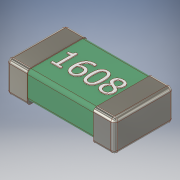
# Autodesk Inventor part: Resistor_1608-0.5mm
Saved by Autodesk Inventor 2018 (Build 220112000, 112)
## iProperties
Created: 2016-08-15
Part Number: Resistor_1608-0.5mm
Material: Copper
Document SubType Name: Modeling
Designer: Bradley
Density: 8.94 g/cm^3
Appearance: Copper - Satin
Author: Bradley
Autodesk Inventor part; units mm, degrees
ref_plane "YZ Plane" through (0, 0, 0) normal (1, 0, 0) x (0, 1, 0)
ref_plane "XZ Plane" through (0, 0, 0) normal (0, 1, 0) x (-1, 0, 0)
ref_plane "XY Plane" through (0, 0, 0) normal (0, 0, 1) x (1, 0, 0)
sketch "Sketch1" plane through (0, 0, 0) normal (0, 0, 1) x (1, 0, 0)
  line L0 (-0.775, 0.4) -> (-0.475, 0.4)
  line L1 (-0.475, 0.4) -> (-0.475, -0.05)
  line L2 (-0.475, -0.05) -> (-0.775, -0.05)
  line L3 (-0.775, -0.05) -> (-0.775, 0.4)
  line L4 (-0.475, 0.39) -> (0.475, 0.39)
  line L5 (0.475, 0.39) -> (0.475, 0)
  line L6 (0.475, 0) -> (-0.475, 0)
  line L7 (-0.475, 0) -> (-0.475, 0.39)
  line L8 (0.475, 0.4) -> (0.775, 0.4)
  line L9 (0.775, 0.4) -> (0.775, -0.05)
  line L10 (0.775, -0.05) -> (0.475, -0.05)
  line L11 (0.475, -0.05) -> (0.475, 0.4)
  point P0 (0, 0)
  point P1 (0, 0.39)
  point P2 (0, 0)
  dimension "d0" = 1.55
  dimension "d1" = 0.45
  dimension "d2" = 0.3
  dimension "d3" = 0.05
  dimension "d6" = 0.01
  constraints: 24 end point, 6 parallel, 3 horizontal, 3 perpendicular, 3 point on line, 2 collinear, 2 midpoint, 1 coincident, 1 vertical alignment
  measures "d0" distance between parallel lines of L9 L3
  measures "d1" distance of L2.end L0.start
  measures "d2" distance of L1.end L2.end
  measures "d3" distance between parallel lines of L2 L6
  measures "d6" distance between parallel lines of L4 L0
extrude "Extrusion1" add sketch "Sketch1" along normal mid plane 0.85 contours L0 L1 L2 L3 | L11 L8 L9 L10 L5
extrude "Extrusion2" add sketch "Sketch1" along normal mid plane 0.84 contours L4 L5 L6 L1
sketch "Sketch3" plane through (-0.475, 0.39, 0.42) normal (0, 1, 0) x (1, 0, 0)
  line L0 (0, 0) -> (0, 0.84) projected
  line L1 (0.95, 0) -> (0, 0) projected
  line L2 (0.95, 0.84) -> (0.95, 0) projected
  line L3 (0, 0.84) -> (0.95, 0.84) projected
  line L4 (0.95, 0.845) -> (0.95, -0.005) construction
  line L5 (0.95, 0.2582) -> (0, 0.2582) construction
  line L6 (0, 0.845) -> (0, -0.005) construction
  line L7 (0.2166, 0.2582) -> (0.0702, 0.2582)
  line L8 (0.0702, 0.2582) -> (0.0702, 0.2888)
  line L9 (0.0702, 0.2888) -> (0.1247, 0.2888)
  line L10 (0.1247, 0.2888) -> (0.1247, 0.4899)
  line L11 (0.1247, 0.4899) -> (0.0702, 0.4899)
  line L12 (0.0702, 0.4899) -> (0.0702, 0.5174)
  spline S0 degree 2 poles (0.0702, 0.5174) (0.1011, 0.5174) (0.1303, 0.5349) (0.1322, 0.5592) knots 0 0 0 1 2 2 2
  line L13 (0.1322, 0.5592) -> (0.1633, 0.5592)
  line L14 (0.1633, 0.5592) -> (0.1633, 0.2888)
  line L15 (0.1633, 0.2888) -> (0.2166, 0.2888)
  line L16 (0.2166, 0.2888) -> (0.2166, 0.2582)
  spline S1 degree 2 poles (0.4614, 0.3555) (0.4614, 0.3324) (0.4461, 0.2932) (0.4332, 0.2801) knots 0 0 0 1 2 2 2
  spline S2 degree 2 poles (0.4332, 0.2801) (0.4198, 0.2662) (0.3863, 0.2519) (0.3661, 0.2519) knots 0 0 0 1 2 2 2
  spline S3 degree 2 poles (0.3661, 0.2519) (0.3459, 0.2519) (0.3126, 0.2655) (0.3, 0.2791) knots 0 0 0 1 2 2 2
  spline S4 degree 2 poles (0.3, 0.2791) (0.2844, 0.2954) (0.2669, 0.3501) (0.2669, 0.39) knots 0 0 0 1 2 2 2
  spline S5 degree 2 poles (0.2669, 0.39) (0.2669, 0.4291) (0.2829, 0.4921) (0.2997, 0.5154) knots 0 0 0 1 2 2 2
  spline S6 degree 2 poles (0.2997, 0.5154) (0.316, 0.5383) (0.3675, 0.5638) (0.4013, 0.5638) knots 0 0 0 1 2 2 2
  spline S7 degree 2 poles (0.4013, 0.5638) (0.4113, 0.5638) (0.4288, 0.5619) (0.4354, 0.5597) knots 0 0 0 1 2 2 2
  line L17 (0.4354, 0.5597) -> (0.4354, 0.521)
  line L18 (0.4354, 0.521) -> (0.4337, 0.521)
  spline S8 degree 2 poles (0.4337, 0.521) (0.4281, 0.5239) (0.4077, 0.529) (0.396, 0.529) knots 0 0 0 1 2 2 2
  spline S9 degree 2 poles (0.396, 0.529) (0.3585, 0.529) (0.3126, 0.4785) (0.3082, 0.4289) knots 0 0 0 1 2 2 2
  spline S10 degree 2 poles (0.3082, 0.4289) (0.3226, 0.4388) (0.3527, 0.4498) (0.3707, 0.4498) knots 0 0 0 1 2 2 2
  spline S11 degree 2 poles (0.3707, 0.4498) (0.3882, 0.4498) (0.4145, 0.4427) (0.4288, 0.432) knots 0 0 0 1 2 2 2
  spline S12 degree 2 poles (0.4288, 0.432) (0.4453, 0.4196) (0.4614, 0.3812) (0.4614, 0.3555) knots 0 0 0 1 2 2 2
  spline S13 degree 2 poles (0.4205, 0.3537) (0.4205, 0.3722) (0.4108, 0.3973) (0.4001, 0.406) knots 0 0 0 1 2 2 2
  spline S14 degree 2 poles (0.4001, 0.406) (0.3921, 0.4123) (0.3722, 0.4165) (0.3617, 0.4165) knots 0 0 0 1 2 2 2
  spline S15 degree 2 poles (0.3617, 0.4165) (0.3476, 0.4165) (0.3211, 0.408) (0.3082, 0.3999) knots 0 0 0 1 2 2 2
  spline S16 degree 2 poles (0.3082, 0.3999) (0.308, 0.3956) (0.3075, 0.3873) (0.3075, 0.381) knots 0 0 0 1 2 2 2
  spline S17 degree 2 poles (0.3075, 0.381) (0.3075, 0.3499) (0.3197, 0.3117) (0.3289, 0.3017) knots 0 0 0 1 2 2 2
  spline S18 degree 2 poles (0.3289, 0.3017) (0.3374, 0.2922) (0.3559, 0.2847) (0.3663, 0.2847) knots 0 0 0 1 2 2 2
  spline S19 degree 2 poles (0.3663, 0.2847) (0.3906, 0.2847) (0.4205, 0.3192) (0.4205, 0.3537) knots 0 0 0 1 2 2 2
  spline S20 degree 2 poles (0.6836, 0.4082) (0.6836, 0.3275) (0.6367, 0.2519) (0.5878, 0.2519) knots 0 0 0 1 2 2 2
  spline S21 degree 2 poles (0.5878, 0.2519) (0.5382, 0.2519) (0.4918, 0.329) (0.4918, 0.408) knots 0 0 0 1 2 2 2
  spline S22 degree 2 poles (0.4918, 0.408) (0.4918, 0.4892) (0.5387, 0.5643) (0.5878, 0.5643) knots 0 0 0 1 2 2 2
  spline S23 degree 2 poles (0.5878, 0.5643) (0.6372, 0.5643) (0.6836, 0.4865) (0.6836, 0.4082) knots 0 0 0 1 2 2 2
  spline S24 degree 2 poles (0.6321, 0.3168) (0.6379, 0.3316) (0.6427, 0.3773) (0.6427, 0.4082) knots 0 0 0 1 2 2 2
  spline S25 degree 2 poles (0.6427, 0.4082) (0.6427, 0.4391) (0.6379, 0.4845) (0.6318, 0.4999) knots 0 0 0 1 2 2 2
  spline S26 degree 2 poles (0.6318, 0.4999) (0.6257, 0.5152) (0.6046, 0.531) (0.5878, 0.531) knots 0 0 0 1 2 2 2
  spline S27 degree 2 poles (0.5878, 0.531) (0.571, 0.531) (0.5494, 0.5152) (0.5431, 0.4994) knots 0 0 0 1 2 2 2
  spline S28 degree 2 poles (0.5431, 0.4994) (0.537, 0.4841) (0.5326, 0.4374) (0.5326, 0.408) knots 0 0 0 1 2 2 2
  spline S29 degree 2 poles (0.5326, 0.408) (0.5326, 0.3764) (0.5365, 0.3341) (0.5428, 0.3175) knots 0 0 0 1 2 2 2
  spline S30 degree 2 poles (0.5428, 0.3175) (0.5487, 0.302) (0.5703, 0.2852) (0.5878, 0.2852) knots 0 0 0 1 2 2 2
  spline S31 degree 2 poles (0.5878, 0.2852) (0.6043, 0.2852) (0.626, 0.301) (0.6321, 0.3168) knots 0 0 0 1 2 2 2
  spline S32 degree 2 poles (0.8127, 0.2514) (0.7903, 0.2514) (0.7536, 0.2648) (0.7407, 0.2772) knots 0 0 0 1 2 2 2
  spline S33 degree 2 poles (0.7407, 0.2772) (0.7281, 0.2893) (0.715, 0.3224) (0.715, 0.3411) knots 0 0 0 1 2 2 2
  spline S34 degree 2 poles (0.715, 0.3411) (0.715, 0.3654) (0.741, 0.4063) (0.7658, 0.4184) knots 0 0 0 1 2 2 2
  line L19 (0.7658, 0.4184) -> (0.7658, 0.4196)
  spline S35 degree 2 poles (0.7658, 0.4196) (0.7436, 0.4325) (0.7222, 0.4631) (0.7222, 0.486) knots 0 0 0 1 2 2 2
  spline S36 degree 2 poles (0.7222, 0.486) (0.7222, 0.5198) (0.7733, 0.565) (0.8127, 0.565) knots 0 0 0 1 2 2 2
  spline S37 degree 2 poles (0.8127, 0.565) (0.8535, 0.565) (0.9029, 0.5222) (0.9029, 0.4887) knots 0 0 0 1 2 2 2
  spline S38 degree 2 poles (0.9029, 0.4887) (0.9029, 0.4685) (0.8793, 0.4291) (0.8572, 0.4179) knots 0 0 0 1 2 2 2
  line L20 (0.8572, 0.4179) -> (0.8572, 0.4167)
  spline S39 degree 2 poles (0.8572, 0.4167) (0.8834, 0.4046) (0.9104, 0.3696) (0.9104, 0.3418) knots 0 0 0 1 2 2 2
  spline S40 degree 2 poles (0.9104, 0.3418) (0.9104, 0.3034) (0.8545, 0.2514) (0.8127, 0.2514) knots 0 0 0 1 2 2 2
  spline S41 degree 2 poles (0.8691, 0.3379) (0.8691, 0.3564) (0.8545, 0.3783) (0.8338, 0.3895) knots 0 0 0 1 2 2 2
  spline S42 degree 2 poles (0.8338, 0.3895) (0.827, 0.3934) (0.8042, 0.4024) (0.7898, 0.4082) knots 0 0 0 1 2 2 2
  spline S43 degree 2 poles (0.7898, 0.4082) (0.7733, 0.3973) (0.7556, 0.3647) (0.7556, 0.344) knots 0 0 0 1 2 2 2
  spline S44 degree 2 poles (0.7556, 0.344) (0.7556, 0.3168) (0.7884, 0.2813) (0.8132, 0.2813) knots 0 0 0 1 2 2 2
  spline S45 degree 2 poles (0.8132, 0.2813) (0.8385, 0.2813) (0.8691, 0.3117) (0.8691, 0.3379) knots 0 0 0 1 2 2 2
  spline S46 degree 2 poles (0.8635, 0.4882) (0.8635, 0.5084) (0.8365, 0.5354) (0.8124, 0.5354) knots 0 0 0 1 2 2 2
  spline S47 degree 2 poles (0.8124, 0.5354) (0.7906, 0.5354) (0.7626, 0.5113) (0.7626, 0.4906) knots 0 0 0 1 2 2 2
  spline S48 degree 2 poles (0.7626, 0.4906) (0.7626, 0.4758) (0.7769, 0.4551) (0.7913, 0.4469) knots 0 0 0 1 2 2 2
  spline S49 degree 2 poles (0.7913, 0.4469) (0.7974, 0.4435) (0.8231, 0.4315) (0.8336, 0.4281) knots 0 0 0 1 2 2 2
  spline S50 degree 2 poles (0.8336, 0.4281) (0.8511, 0.4415) (0.8635, 0.47) (0.8635, 0.4882) knots 0 0 0 1 2 2 2
  point P0 (0.475, 0.42)
  constraints: 2 end point, 2 point on line, 1 horizontal, 1 perpendicular
extrude "Extrusion4" add sketch "Sketch3" along normal blind 0.01 contours L7 L8 L9 L10 L11 L12 S0 L13 L14 L15 L16 | S20 S21 S22 S23 | S32 S33 S34 S35 S36 S37 S38 S39 S40
fillet "Fillet1" radius 0.05 20 edges at (-0.625, 0.4, 0.425) (0, 0.39, 0.42) (0.625, 0.4, 0.425) (-0.625, 0.4, -0.425) (0, 0.39, -0.42) (0.625, 0.4, -0.425) (0.775, 0.4, 0) (0.775, 0.175, -0.425) (0.775, -0.05, 0) (0.625, -0.05, -0.425) (0.625, -0.05, 0.425) (0.775, 0.175, 0.425) (0, 0, 0.42) (0, 0, -0.42) (-0.625, -0.05, -0.425) (-0.775, -0.05, 0) (-0.775, 0.175, 0.425) (-0.625, -0.05, 0.425) (-0.775, 0.175, -0.425) (-0.775, 0.4, 0)
body "Solid1"
